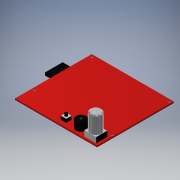
# Autodesk Inventor part: Rød PCB
Saved by Autodesk Inventor 2016 (Build 200138000, 138)
## iProperties
Created: 2015-06-10
Part Number: Rød PCB
Material: Generic
Document SubType Name: Modeling
Designer: Mathias L. Kjeldgaard
Density: 1 g/cm^3
Appearance: Default
Author: Mathias L. Kjeldgaard
Autodesk Inventor part; units mm, degrees
ref_plane "YZ Plane" through (0, 0, 0) normal (1, 0, 0) x (0, 1, 0)
ref_plane "XZ Plane" through (0, 0, 0) normal (0, 1, 0) x (-1, 0, 0)
ref_plane "XY Plane" through (0, 0, 0) normal (0, 0, 1) x (1, 0, 0)
sketch "Sketch1" plane through (0, 0, 0) normal (0, 0, 1) x (1, 0, 0)
  line L0 (-46.5, 43.5) -> (46.5, 43.5)
  line L1 (46.5, 43.5) -> (46.5, -43.5)
  line L2 (46.5, -43.5) -> (-46.5, -43.5)
  line L3 (-46.5, -43.5) -> (-46.5, 43.5)
  point P0 (0, 0)
  dimension "d0" = 93
  dimension "d1" = 87
  dimension "d2" = 46.5
  dimension "d3" = 43.5
  constraints: 8 end point, 2 parallel, 1 horizontal, 1 perpendicular
  measures "d0" distance of L1.end L2.end
  measures "d1" distance of L0.end L1.end
  measures "d2" distance from line of L1 point (0, 0)
  measures "d3" distance from line of L0 point (0, 0)
extrude "Tykkelse Rød PCB" add sketch "Sketch1" along normal blind 1.5
sketch "Sketch2" plane through (0, 0, 1.5) normal (0, 0, 1) x (1, 0, 0)
  line L0 (46.5, 43.5) -> (-46.5, 43.5) projected
  line L1 (-46.5, 43.5) -> (-46.5, -43.5) projected
  line L2 (46.5, -43.5) -> (46.5, 43.5) projected
  circle A0 centre (44, 41) radius 1.5
  circle A1 centre (-44, 41) radius 1.5
  line L3 (45.5, 42.5) -> (45.5, 26.8687) construction
  line L4 (4.2035, 42.5) -> (45.5, 42.5) construction
  line L5 (-45.5, 42.5) -> (-9.5739, 42.5) construction
  line L6 (-45.5, 42.5) -> (-45.5, 29.332) construction
  line L7 (-46.5, -43.5) -> (46.5, -43.5) projected
  circle A2 centre (-44, -24) radius 1.5
  circle A3 centre (44, -24) radius 1.5
  line L8 (45.5, -14.3819) -> (45.5, -25.5) construction
  line L9 (45.5, -25.5) -> (38.4616, -25.5) construction
  line L10 (-45.5, -14.3819) -> (-45.5, -25.5) construction
  line L11 (-36.8227, -25.5) -> (-45.5, -25.5) construction
  point P0 (0, 0)
  dimension "d6" = 3
  dimension "d7" = 3
  dimension "d8" = 1
  dimension "d9" = 1
  dimension "d10" = 1
  dimension "d11" = 1
  dimension "d79" = 1
  dimension "d80" = 3
  dimension "d81" = 65
  dimension "d82" = 3
  dimension "d83" = 1
  dimension "d84" = 65
  constraints: 16 end point, 8 tangent, 6 perpendicular, 4 centre point, 2 parallel, 1 collinear
  measures "d6" diameter of A0
  measures "d7" diameter of A1
  measures "d8" distance between parallel lines of L0 L5
  measures "d9" distance between parallel lines of L0 L4
  measures "d10" distance between parallel lines of L2 L3
  measures "d11" distance between parallel lines of L1 L6
  measures "d79" distance between parallel lines of L1 L10
  measures "d80" diameter of A2
  measures "d81" distance of A1.centre A2.centre
  measures "d82" diameter of A3
  measures "d83" distance between parallel lines of L2 L8
  measures "d84" distance of A0.centre A3.centre
extrude "Monteringshuller Ø3" cut sketch "Sketch2" against normal up to surface (1.5 mm away) contours A0 | A1 | A2 | A3
sketch "Sketch3" plane through (0, 0, 0) normal (0, 0, -1) x (-1, 0, 0)
  line L0 (46.5, 43.5) -> (-46.5, 43.5) projected
  line L1 (-46.5, 43.5) -> (-46.5, -43.5) projected
  line L2 (46.5, -43.5) -> (46.5, 43.5) projected
  line L3 (-25.5, 37.5) -> (-5.5, 37.5)
  line L4 (-5.5, 37.5) -> (-5.5, 28.5)
  line L5 (-5.5, 28.5) -> (-25.5, 28.5)
  line L6 (-25.5, 28.5) -> (-25.5, 37.5)
  line L7 (5.5, 37.5) -> (25.5, 37.5)
  line L8 (25.5, 37.5) -> (25.5, 28.5)
  line L9 (25.5, 28.5) -> (5.5, 28.5)
  line L10 (5.5, 28.5) -> (5.5, 37.5)
  point P0 (0, 0)
  dimension "d14" = 20
  dimension "d15" = 9
  dimension "d16" = 9
  dimension "d17" = 20
  dimension "d18" = 21
  dimension "d19" = 21
  dimension "d20" = 6
  dimension "d21" = 6
  constraints: 16 end point, 4 parallel, 2 horizontal, 2 perpendicular
  measures "d14" distance of L8.end L9.end
  measures "d15" distance of L7.end L8.end
  measures "d16" distance of L3.end L4.end
  measures "d17" distance of L4.end L5.end
  measures "d18" distance between parallel lines of L2 L8
  measures "d19" distance between parallel lines of L1 L6
  measures "d20" distance between parallel lines of L0 L7
  measures "d21" distance between parallel lines of L0 L3
extrude "Sorte Stik" add sketch "Sketch3" along normal blind 9
sketch "Sketch4" plane through (0, 0, 0) normal (0, 0, -1) x (-1, 0, 0)
  line L0 (46.5, 43.5) -> (-46.5, 43.5) projected
  line L1 (46.5, -43.5) -> (46.5, 43.5) projected
  line L2 (25.5, 21.5) -> (46.5, 21.5)
  line L3 (46.5, 21.5) -> (46.5, -0.5)
  line L4 (46.5, -0.5) -> (25.5, -0.5)
  line L5 (25.5, -0.5) -> (25.5, 21.5)
  point P0 (0, 0)
  dimension "d24" = 22
  dimension "d25" = 21
  dimension "d26" = 0
  dimension "d27" = 22
  constraints: 8 end point, 2 parallel, 1 horizontal, 1 perpendicular
  measures "d24" distance of L4.end L2.start
  measures "d25" distance of L3.end L4.end
  measures "d26" distance between parallel lines of L1 L3
  measures "d27" distance between parallel lines of L0 L2
extrude "SD Kort læser" add sketch "Sketch4" along normal blind 4
sketch "Sketch5" plane through (0, 0, 1.5) normal (0, 0, 1) x (1, 0, 0)
  line L0 (-46.5, -43.5) -> (46.5, -43.5) projected
  line L1 (46.5, -43.5) -> (46.5, 43.5) projected
  line L2 (43.5, -29) -> (30, -29)
  line L3 (30, -29) -> (30, -41.5)
  line L4 (30, -41.5) -> (43.5, -41.5)
  line L5 (43.5, -41.5) -> (43.5, -29)
  point P0 (0, 0)
  dimension "d30" = 12.5
  dimension "d31" = 13.5
  dimension "d32" = 3
  dimension "d33" = 2
  constraints: 8 end point, 2 parallel, 1 horizontal, 1 perpendicular
  measures "d30" distance of L2.end L3.end
  measures "d31" distance between parallel lines of L3 L5
  measures "d32" distance between parallel lines of L1 L5
  measures "d33" distance between parallel lines of L0 L4
extrude "Extrusion5" add sketch "Sketch5" along normal blind 6
sketch "Sketch6" plane through (0, 0, 7.5) normal (0, 0, 1) x (1, 0, 0)
  line L0 (43.5, -29) -> (30, -29) projected
  line L1 (30, -29) -> (30, -41.5) projected
  line L2 (30, -41.5) -> (43.5, -41.5) projected
  circle A0 centre (36.75, -35.25) radius 6.25
  point P0 (0, 0)
  dimension "d36" = 6.75
  dimension "d37" = 13.5
  constraints: 2 tangent, 1 centre point
  measures "d36" distance from line of L1 A0.centre
  measures "d37" distance of L0.start L0.end
extrude "Extrusion6" add sketch "Sketch6" along normal blind 19 contours A0
chamfer "Chamfer1" distance 1 angle 45 1 edges at (30.5, -35.25, 26.5)
sketch "Sketch7" plane through (0, 0, 1.5) normal (0, 0, 1) x (1, 0, 0)
  line L0 (-46.5, -43.5) -> (46.5, -43.5) projected
  line L1 (46.5, -43.5) -> (46.5, 43.5) projected
  circle A0 centre (19.75, -34.75) radius 5.75
  line L2 (25.5, -40.5) -> (6.0957, -40.5) construction
  line L3 (25.5, -23.1538) -> (25.5, -40.5) construction
  point P0 (0, 0)
  dimension "d43" = 11.5
  dimension "d44" = 3
  dimension "d45" = 21
  constraints: 4 end point, 2 perpendicular, 2 tangent, 1 centre point
  measures "d43" diameter of A0
  measures "d44" distance between parallel lines of L0 L2
  measures "d45" distance between parallel lines of L1 L3
extrude "Extrusion7" add sketch "Sketch7" along normal blind 9
sketch "Sketch8" plane through (19.75, -34.75, 10.5) normal (0, 0, 1) x (1, 0, 0)
  circle A0 centre (0, 0) radius 5.75 projected
  circle A1 centre (0, 0) radius 1
  point P0 (-19.75, 34.75)
  dimension "d48" = 2
  constraints: 1 centre point, 1 coincident
  measures "d48" diameter of A1
extrude "Extrusion8" cut sketch "Sketch8" against normal blind 4 contours A1
sketch "Sketch9" plane through (0, 0, 1.5) normal (0, 0, 1) x (1, 0, 0)
  line L0 (-46.5, -43.5) -> (46.5, -43.5) projected
  line L1 (46.5, -43.5) -> (46.5, 43.5) projected
  line L2 (0.5, -32.5) -> (6.5, -32.5)
  line L3 (6.5, -32.5) -> (6.5, -38.5)
  line L4 (6.5, -38.5) -> (0.5, -38.5)
  line L5 (0.5, -38.5) -> (0.5, -32.5)
  point P0 (0, 0)
  dimension "d51" = 6
  dimension "d52" = 6
  dimension "d53" = 5
  dimension "d54" = 40
  constraints: 8 end point, 2 parallel, 1 horizontal, 1 perpendicular
  measures "d51" distance of L2.end L3.end
  measures "d52" distance between parallel lines of L5 L3
  measures "d53" distance between parallel lines of L0 L4
  measures "d54" distance between parallel lines of L1 L3
extrude "Extrusion9" add sketch "Sketch9" along normal blind 4
sketch "Sketch10" plane through (0, 0, 5.5) normal (0, 0, 1) x (1, 0, 0)
  line L0 (6.5, -32.5) -> (0.5, -32.5) projected
  line L1 (6.5, -38.5) -> (6.5, -32.5) projected
  circle A0 centre (3.5, -35.5) radius 1.5
  point P0 (0, 0)
  dimension "d57" = 3
  dimension "d58" = 6
  dimension "d59" = 6
  dimension "d60" = 3
  dimension "d61" = 3
  constraints: 1 centre point
  measures "d57" diameter of A0
  measures "d58" distance of L1.start L0.start
  measures "d59" distance of L0.start L0.end
  measures "d60" distance from line of L0 A0.centre
  measures "d61" distance from line of L1 A0.centre
extrude "Extrusion10" add sketch "Sketch10" along normal blind 3
fillet "Fillet1" radius 0.5 1 edges at (2, -35.5, 8.5)
fillet "Fillet2" radius 0.5 1 edges at (14, -34.75, 10.5)
sketch "Sketch11" plane through (36.75, -35.25, 26.5) normal (0, 0, 1) x (1, 0, 0)
  circle A0 centre (0, 0) radius 5.25 projected
  line L0 (0, 0) -> (0, -4.739) construction
  line L1 (0, 0) -> (-2.5895, -4.4851) construction
  line L2 (-2.089, -3.1183) -> (-3.339, -5.2833)
  line L3 (-2.089, -3.1183) -> (-1.656, -3.3683)
  circle A1 centre (0, 0) radius 6.25 projected
  circle A2 centre (0, 0) radius 5.25 projected
  line L4 (-2.906, -5.5333) -> (-1.656, -3.3683)
  point P0 (-36.75, 35.25)
  dimension "d66" = 30
  dimension "d68" = 0.25
  dimension "d69" = 2.5
  dimension "d70" = 0.5
  constraints: 10 end point, 2 parallel, 2 point on circle, 1 perpendicular, 1 vertical
  measures "d66" angle of L0 L1
  measures "d68" distance between parallel lines of L1 L2
  measures "d69" distance from line of L4.start L3
  measures "d70" distance between parallel lines of L2 L4
extrude "Extrusion11" cut sketch "Sketch11" against normal blind 1 contours L2 L3 L4 A0 | A0 L4 A1 L2 picked at (-2.0992, -3.6914) picked at (-2.6213, -4.9292)
sketch "Sketch12" plane through (-46.5, -43.5, 1.5) normal (-1, 0, 0) x (0, 0, 1)
  line L0 (-1.5, 65) -> (-1.5, 87) projected
  line L1 (-1.5, 65) -> (-5.5, 65) projected
  line L2 (-5.5, 43) -> (-5.5, 65) projected
  line L3 (-1.5, 43) -> (-5.5, 43) projected
  line L4 (-4.5, 64) -> (-1.5, 64)
  line L5 (-1.5, 64) -> (-1.5, 44)
  line L6 (-1.5, 44) -> (-4.5, 44)
  line L7 (-4.5, 44) -> (-4.5, 64)
  point P0 (-1.5, 43.5)
  dimension "d73" = 1
  dimension "d74" = 1
  dimension "d75" = 1
  dimension "d76" = 0
  constraints: 8 end point, 2 parallel, 1 horizontal, 1 perpendicular
  measures "d73" distance between parallel lines of L3 L6
  measures "d74" distance between parallel lines of L1 L4
  measures "d75" distance between parallel lines of L2 L7
  measures "d76" distance between parallel lines of L0 L5
extrude "Extrusion12" add sketch "Sketch12" along normal blind 10
sketch "Sketch13" plane through (0, 0, 26.5) normal (0, 0, 1) x (1, 0, 0)
  arc A0 (-34.5, 28.5) -> (-36.5, 26.5) centre (-34.5, 26.5) ccw projected
  line L0 (-34.5, 28.5) -> (34.5, 28.5) projected
  arc A1 (36.5, 26.5) -> (34.5, 28.5) centre (34.5, 26.5) ccw projected
  line L1 (36.5, 26.5) -> (36.5, -8.5) projected
  arc A2 (34.5, -10.5) -> (36.5, -8.5) centre (34.5, -8.5) ccw projected
  line L2 (34.5, -10.5) -> (-34.5, -10.5) projected
  arc A3 (-36.5, -8.5) -> (-34.5, -10.5) centre (-34.5, -8.5) ccw projected
  line L3 (-36.5, -8.5) -> (-36.5, 26.5) projected
  line L4 (39, 34.5) -> (-39, 34.5) projected
  line L5 (-39, 34.5) -> (-39, -16.5) projected
  line L6 (-39, -16.5) -> (39, -16.5) projected
  line L7 (39, -16.5) -> (39, 34.5) projected
  line L8 (-39, 30.5) -> (-39, -11.5) projected
  line L9 (-39, 30.5) -> (-45.5, 30.5) projected
  line L10 (-45.5, 30.5) -> (-45.5, -11.5) projected
  line L11 (-45.5, -11.5) -> (-39, -11.5) projected
  circle A4 centre (3.5, -35.5) radius 1.5 projected
  circle A5 centre (19.75, -34.75) radius 5.75 projected
  arc A6 (33.844, -40.7833) -> (33.411, -40.5333) centre (36.75, -35.25) ccw projected
  line L12 (-34.5, 26.5) -> (34.5, -8.5) construction
  line L13 (34.5, 26.5) -> (-34.5, -8.5) construction
  line L14 (0, 28.5) -> (0, 9) construction
  point P0 (0, 0)
  dimension "d85" = 36.75
  dimension "d86" = 6.25
  dimension "d87" = 11.5
  dimension "d88" = 19.75
  dimension "d89" = 3
  dimension "d90" = 3.5
  dimension "d91" = 44.5
  dimension "d92" = 43.75
  dimension "d93" = 44.25
  constraints: 6 end point, 2 midpoint
  measures "d85" distance from line of A6.centre L14
  measures "d86" radius of A6
  measures "d87" diameter of A5
  measures "d88" distance from line of A5.centre L14
  measures "d89" diameter of A4
  measures "d90" distance from line of A4.centre L14
  measures "d91" vertical distance of L14.end A4.centre
  measures "d92" vertical distance of L14.end A5.centre
  measures "d93" vertical distance of L14.end A6.centre
equation "\"d2\" = 0.5 * d0"
equation "\"d3\" = 0.5 * d1"
equation "\"d16\" = d15"
equation "\"d17\" = d14"
equation "\"d19\" = d18"
equation "\"d21\" = d20"
equation "\"d36\" = 0.5 * d37"
equation "\"d60\" = 0.5 * d58"
equation "\"d61\" = 0.5 * d59"
equation "\"d68\" = 0.5 * d70"
body "Solid1"
